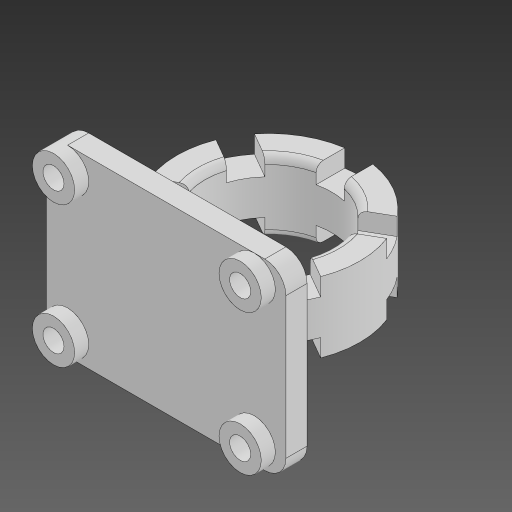
# Autodesk Inventor part: Ind_1
Saved by Autodesk Inventor 2023.2 (Build 272271000, 271)
## iProperties
Created: 2023-04-07
Part Number: Ind_1
Material: Generic
Document SubType Name: Modeling
Designer: jcgg2
Density: 1 g/cm^3
Appearance: Default
Mass: 4.97039 g
Surface Area: 39.7774 cm^2
Volume: 4.97039 cm^3
Author: jcgg2
Autodesk Inventor part; units mm, degrees
ref_plane "YZ Plane" through (0, 0, 0) normal (1, 0, 0) x (0, 1, 0)
sketch "Sketch1" plane through (0, 0, 0) normal (0, 1, 0) x (-1, 0, 0)
  circle A0 centre (0, 0) radius 9
  circle A1 centre (0, 0) radius 13
  dimension "d0" = 18
  dimension "d1" = 4
  constraints: 2 centre point, 1 coincident
  measures "d0" diameter of A0
  measures "d1" radial gap between concentric circles of A0 A1
extrude "Extrusion1" add sketch "Sketch1" along normal blind 10
ref_plane "Work Plane1" through (0, 0, 13) normal (0, 0, 1) x (1, 0, 0)
sketch "Sketch2" plane through (0, 0, 13) normal (0, 0, 1) x (1, 0, 0)
  line L0 (-17, -8) -> (17, -8)
  line L1 (17, -8) -> (17, 18)
  line L2 (17, 18) -> (-17, 18)
  line L3 (-17, 18) -> (-17, -8)
  point P0 (0, 0)
  point P1 (-14, -5)
  point P2 (-14, 15)
  point P3 (12.5, 15)
  point P4 (12.5, -5)
  dimension "d5" = 34
  dimension "d6" = 26
  dimension "d7" = 20
  dimension "d8" = 26.5
  dimension "d9" = 3
  dimension "d10" = 3
  dimension "d11" = 17
  dimension "d12" = 8
  constraints: 8 end point, 2 horizontal alignment, 2 parallel, 2 vertical alignment, 1 horizontal, 1 perpendicular
  measures "d5" distance of L2.end L1.end
  measures "d6" distance of L1.end L0.end
  measures "d7" distance of point (-14, 15) point (-14, -5)
  measures "d8" distance of point (-14, -5) point (12.5, -5)
  measures "d9" distance from line of L0 point (-14, -5)
  measures "d10" distance from line of L3 point (-14, -5)
  measures "d11" distance from line of L3 point (0, 0)
  measures "d12" distance from line of L0 point (0, 0)
extrude "Extrusion2" add sketch "Sketch2" along normal mid plane 3
hole "Hole1" at (-14, -5, 13) at (-14, 15, 13) at (12.5, 15, 13) at (12.5, -5, 13) direction (0, 0, 1) diameter 3 depth 12
hole "Hole2" at (-14, -5, 13) at (-14, 15, 13) at (12.5, 15, 13) at (12.5, -5, 13) direction (0, 0, -1) diameter 3 depth 12
fillet "Fillet1" radius 3 4 edges at (-17, -8, 13) (-17, 18, 13) (17, 18, 13) (17, -8, 13)
sketch "Sketch3" plane through (0, 10, 0) normal (0, 1, 0) x (1, 0, 0)
  line L0 (0, 0) -> (0, 20.083) construction
  line L1 (-2, 8) -> (2, 8)
  line L2 (2, 8) -> (2, 14)
  line L3 (2, 14) -> (-2, 14)
  line L4 (-2, 14) -> (-2, 8)
  dimension "d30" = 4
  dimension "d31" = 6
  dimension "d32" = 2
  dimension "d33" = 8
  constraints: 10 end point, 2 parallel, 1 horizontal, 1 perpendicular, 1 vertical
  measures "d30" distance of L3.end L2.end
  measures "d31" distance of L2.end L1.end
  measures "d32" distance between parallel lines of L4 L0
  measures "d33" distance from line of L0.start L1
extrude "Extrusion3" cut sketch "Sketch3" against normal blind 2.5
pattern_circular "Circular Pattern1" count 6 over 360 about axis through (0, 0, 0) along (0, 1, 0) of "Extrusion3"
ref_plane "Work Plane2" through (0, 5, 0) normal (0, 1, 0) x (1, 0, 0)
mirror "Mirror1" about plane through (0, 5, 0) normal (0, 1, 0) of "Extrusion3", "Circular Pattern1"
fillet "Fillet2" radius 2 6 edges at (4.0311, 10, 11.5) (-4.0311, 10, 11.5) (-6.0622, 5, 11.5) (6.0622, 5, 11.5) (4.0311, 0, 11.5) (-4.0311, 0, 11.5)
fillet "Fillet3" radius 1 14 edges at (-4.5, 10, 7.7942) (-8.8993, 10, -1.3427) (-8.8993, 10, 1.3427) (-4.5, 10, -7.7942) (4.5, 10, -7.7942) (9, 10, 0) (4.5, 10, 7.7942) (-4.5, 0, -7.7942) (-8.8993, 0, 1.3427) (-8.8993, 0, -1.3427) (4.5, 0, -7.7942) (9, 0, 0) (4.5, 0, 7.7942) (-4.5, 0, 7.7942)
sketch "Sketch4" plane through (0, 0, 14.5) normal (0, 0, 1) x (1, 0, 0)
  arc A0 (14, -8) -> (17, -5) centre (14, -5) ccw projected
  line L0 (17, -5) -> (17, 15) projected
  arc A1 (17, 15) -> (14, 18) centre (14, 15) ccw projected
  line L1 (14, 18) -> (-14, 18) projected
  arc A2 (-14, 18) -> (-17, 15) centre (-14, 15) ccw projected
  line L2 (-17, 15) -> (-17, -5) projected
  arc A3 (-17, -5) -> (-14, -8) centre (-14, -5) ccw projected
  line L3 (-14, -8) -> (14, -8) projected
  circle A4 centre (12.5, 15) radius 1.5 projected
  circle A5 centre (-14, -5) radius 1.5 projected
  circle A6 centre (-14, 15) radius 1.5 projected
  circle A7 centre (12.5, -5) radius 1.5 projected
  circle A8 centre (-14, -5) radius 3
  circle A9 centre (-14, 15) radius 3
  circle A10 centre (12.5, 15) radius 3
  circle A11 centre (12.5, -5) radius 3
  point P0 (0, 0)
  dimension "d42" = 1.5
  dimension "d43" = 1.5
  dimension "d44" = 1.5
  dimension "d45" = 1.5
  constraints: 4 centre point
  measures "d42" radial gap between concentric circles of A5 A8
  measures "d43" radial gap between concentric circles of A6 A9
  measures "d44" radial gap between concentric circles of A4 A10
  measures "d45" radial gap between concentric circles of A7 A11
extrude "Extrusion4" add sketch "Sketch4" along normal blind 2 contours A10 | A11 | A3 A8 | A2 A9
equation "\"d0\" = fing_diam"
equation "\"fing_diam\" = 18"
body "Solid1"
